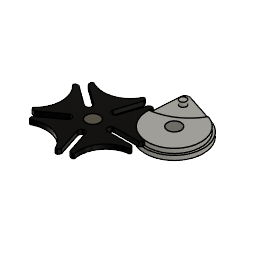
GenevaMechanism (Autodesk Fusion 360 design; units mm, degrees)
part number: 2026-03-22-09-52-00-006
part number: 2026-03-22-09-52-33-959
part number: 2026-03-22-10-12-23-984
part number: 2026-03-22-10-22-25-082
part number: 2026-03-23-03-52-01-189
Autodesk Fusion 360 part; units mm, degrees
sketch "Sketch1" plane through (0, 0, 0) normal (0, 0, 1) x (1, 0, 0) in component "Follower"
  circle A0 centre (0, 0) radius 7.5
  circle A1 centre (0, 0) radius 50
  line L0 (20, -3.75) -> (60, -3.75)
  arc A2 (60, -3.75) -> (60, 3.75) centre (60, 0) ccw
  line L1 (60, 3.75) -> (20, 3.75)
  arc A3 (20, 3.75) -> (20, -3.75) centre (20, 0) ccw
  line L2 (20, 0) -> (60, 0) construction
  line L3 (14.9746, 58.2222) -> (2.6139, 20.1799)
  arc A4 (2.6139, 20.1799) -> (9.7468, 17.8623) centre (6.1803, 19.0211) ccw
  line L4 (9.7468, 17.8623) -> (22.1075, 55.9046)
  arc A5 (22.1075, 55.9046) -> (14.9746, 58.2222) centre (18.541, 57.0634) ccw
  line L5 (-50.7452, 32.2333) -> (-18.3845, 8.7219)
  arc A6 (-18.3845, 8.7219) -> (-13.9761, 14.7895) centre (-16.1803, 11.7557) ccw
  line L6 (-13.9761, 14.7895) -> (-46.3368, 38.3009)
  arc A7 (-46.3368, 38.3009) -> (-50.7452, 32.2333) centre (-48.541, 35.2671) ccw
  line L7 (-46.3368, -38.3009) -> (-13.9761, -14.7895)
  arc A8 (-13.9761, -14.7895) -> (-18.3845, -8.7219) centre (-16.1803, -11.7557) ccw
  line L8 (-18.3845, -8.7219) -> (-50.7452, -32.2333)
  arc A9 (-50.7452, -32.2333) -> (-46.3368, -38.3009) centre (-48.541, -35.2671) ccw
  line L9 (22.1075, -55.9046) -> (9.7468, -17.8623)
  arc A10 (9.7468, -17.8623) -> (2.6139, -20.1799) centre (6.1803, -19.0211) ccw
  line L10 (2.6139, -20.1799) -> (14.9746, -58.2222)
  arc A11 (14.9746, -58.2222) -> (22.1075, -55.9046) centre (18.541, -57.0634) ccw
  circle A12 centre (52.5861, 38.206) radius 30
  line L11 (52.5861, 38.206) -> (20, 0) construction
  line L12 (52.5861, 38.206) -> (6.1803, 19.0211) construction
  circle A13 centre (-20.0861, 61.8187) radius 30
  circle A14 centre (-65, 0) radius 30
  circle A15 centre (-20.0861, -61.8187) radius 30
  circle A16 centre (52.5861, -38.206) radius 30
  dimension "d12" = 15
  dimension "d13" = 100
  dimension "d14" = 7.5
  dimension "d15" = 20
  dimension "d17" = 360
  dimension "d18" = 60
  dimension "d19" = 65
  dimension "d21" = 360
  constraint coincident A0.centre A1.centre
  constraint tangent L0 A2
  constraint tangent A2 L1
  constraint parallel L0 L1
  constraint tangent L1 A3
  constraint tangent L0 A3
  constraint horizontal L2
  constraint horizontal A0.centre A3.centre
  constraint coincident A12.centre L11.start
  constraint coincident A3.centre L2.start
  constraint coincident A4.centre L12.end
  constraint equal L11 L12
  measures "d12" diameter of A0
  measures "d13" diameter of A1
  measures "d14" diameter of A2
  measures "d15" distance of A0.centre A3.centre
  measures "d18" diameter of A12
  measures "d19" distance of A0.centre A12.centre
extrude "Extrude1" add sketch "Sketch1" along normal blind 5 contours A1 L0 L1 A3 L3 A4 L4 L5 A6 L6 L7 A8 L8 L9 A10 L10 A12 A13 A14 A15 A16 makes body 1 in component "Follower"
chamfer "Chamfer1" distance 2.5 angle 45 10 edges at (11.8409, -48.5777, 2.5) (18.9738, -46.2601, 2.5) (-38.1327, -32.3403, 2.5) (-42.5411, -26.2727, 2.5) (-42.5411, 26.2727, 2.5) (-38.1327, 32.3403, 2.5) (11.8409, 48.5777, 2.5) (18.9738, 46.2601, 2.5) (49.8592, -3.75, 2.5) (49.8592, 3.75, 2.5) on bodies 1 in component "Follower"
sketch "Sketch1 (2)" plane through (0, 0, 5) normal (0, 0, 1) x (-1, 0, 0) in component "FollowJoint"
  line L0 (-47.3592, -3.75) -> (-49.6094, -6.2375)
  arc A0 (-49.6094, -6.2375) -> (-49.2915, -8.3875) centre (0, 0) ccw
  arc A1 (-23.2089, -44.2871) -> (-49.2915, -8.3875) centre (-52.5861, -38.206) ccw
  arc A2 (-23.2089, -44.2871) -> (-21.2624, -45.2539) centre (0, 0) ccw
  line L1 (-21.2624, -45.2539) -> (-18.2013, -43.8824)
  line L2 (-18.2013, -43.8824) -> (-9.7468, -17.8623)
  arc A3 (-2.6139, -20.1799) -> (-9.7468, -17.8623) centre (-6.1803, -19.0211) ccw
  line L3 (-2.6139, -20.1799) -> (-11.0683, -46.2001)
  line L4 (-11.0683, -46.2001) -> (-9.3979, -49.1088)
  arc A4 (-9.3979, -49.1088) -> (-7.2549, -49.4709) centre (0, 0) ccw
  arc A5 (34.9476, -35.7584) -> (-7.2549, -49.4709) centre (20.0861, -61.8187) ccw
  arc A6 (34.9476, -35.7584) -> (36.4686, -34.2059) centre (0, 0) ccw
  line L5 (36.4686, -34.2059) -> (36.1102, -30.8708)
  line L6 (36.1102, -30.8708) -> (13.9761, -14.7895)
  arc A7 (18.3845, -8.7219) -> (13.9761, -14.7895) centre (16.1803, -11.7557) ccw
  line L7 (18.3845, -8.7219) -> (40.5186, -24.8032)
  line L8 (40.5186, -24.8032) -> (43.8012, -24.1134)
  arc A8 (43.8012, -24.1134) -> (44.8077, -22.1872) centre (0, 0) ccw
  arc A9 (44.8077, 22.1872) -> (44.8077, -22.1872) centre (65, 0) ccw
  arc A10 (44.8077, 22.1872) -> (43.8012, 24.1134) centre (0, 0) ccw
  line L9 (43.8012, 24.1134) -> (40.5186, 24.8032)
  line L10 (40.5186, 24.8032) -> (18.3845, 8.7219)
  arc A11 (13.9761, 14.7895) -> (18.3845, 8.7219) centre (16.1803, 11.7557) ccw
  line L11 (13.9761, 14.7895) -> (36.1102, 30.8708)
  line L12 (36.1102, 30.8708) -> (36.4686, 34.2059)
  arc A12 (36.4686, 34.2059) -> (34.9476, 35.7584) centre (0, 0) ccw
  arc A13 (-7.2549, 49.4709) -> (34.9476, 35.7584) centre (20.0861, 61.8187) ccw
  arc A14 (-7.2549, 49.4709) -> (-9.3979, 49.1088) centre (0, 0) ccw
  line L13 (-9.3979, 49.1088) -> (-11.0683, 46.2001)
  line L14 (-11.0683, 46.2001) -> (-2.6139, 20.1799)
  arc A15 (-9.7468, 17.8623) -> (-2.6139, 20.1799) centre (-6.1803, 19.0211) ccw
  line L15 (-9.7468, 17.8623) -> (-18.2013, 43.8824)
  line L16 (-18.2013, 43.8824) -> (-21.2624, 45.2539)
  arc A16 (-21.2624, 45.2539) -> (-23.2089, 44.2871) centre (0, 0) ccw
  arc A17 (-49.2915, 8.3875) -> (-23.2089, 44.2871) centre (-52.5861, 38.206) ccw
  arc A18 (-49.2915, 8.3875) -> (-49.6094, 6.2375) centre (0, 0) ccw
  line L17 (-49.6094, 6.2375) -> (-47.3592, 3.75)
  line L18 (-47.3592, 3.75) -> (-20, 3.75)
  arc A19 (-20, -3.75) -> (-20, 3.75) centre (-20, 0) ccw
  line L19 (-20, -3.75) -> (-47.3592, -3.75)
  circle A20 centre (0, 0) radius 7.5
  circle A21 centre (0, 0) radius 7.5
extrude "Extrude1'" add sketch "Sketch1 (2)" against normal blind 10 separate body contours A20 A21 makes body 2 in component "FollowJoint"
sketch "Sketch1 (3)" plane through (0, 0, 0) normal (0, 0, 1) x (1, 0, 0)
sketch "Sketch1 (4)" plane through (0, 0, 0) normal (0, 0, 1) x (1, 0, 0) in component "Cam"
  circle A0 centre (52.5861, 38.206) radius 7.5
  arc A1 (23.2089, 44.2871) -> (49.2915, 8.3875) centre (52.5861, 38.206) ccw
  line L0 (52.5861, 38.206) -> (158.6521, 144.2721) construction
  line L1 (52.5861, 38.206) -> (202.5861, 38.206) construction
  circle A2 centre (79.1026, 64.7225) radius 3.75
  arc A3 (89.365, 69.3879) -> (83.768, 74.985) centre (84.4059, 70.0258) ccw
  line L2 (83.768, 74.985) -> (48.4396, 70.4404)
  line L3 (89.365, 69.3879) -> (84.8205, 34.0595)
  arc A4 (48.6183, 67.9425) -> (82.3226, 34.2382) centre (98.548, 84.168) ccw
  arc A5 (48.6183, 67.9425) -> (82.3226, 34.2382) centre (52.5861, 38.206) ccw
  arc A6 (48.4396, 70.4404) -> (85.0861, 38.206) centre (52.5861, 38.206) ccw
  dimension "d27" = 65
  dimension "d28" = 60
  dimension "d29" = 15
  dimension "d30" = 150
  dimension "d31" = 45
  dimension "d32" = 7.5
  dimension "d33" = 10
  dimension "d34" = 37.5
  dimension "d35" = 45
  dimension "d36" = 105
  dimension "d37" = 65
  constraint concentric A5 A6
  constraint concentric A0 A5
  constraint tangent A1 A5
  constraint horizontal L1
  constraint coincident A0.centre A1.centre
  constraint coincident L0 A2.centre
  constraint coincident L0 A3.centre
  constraint tangent A3 L2
  constraint tangent L2 A6
  constraint tangent A3 L3
  constraint tangent L3 A6
  constraint coincident L3.end A6
  constraint coincident L0 A4.centre
  constraint coincident L1 A6.end
  measures "d27" diameter of A6
  measures "d28" diameter of A5
  measures "d29" diameter of A0
  measures "d30" distance of A0.centre L0.end
  measures "d31" angle of L0 L1
  measures "d32" diameter of A2
  measures "d33" diameter of A3
  measures "d34" distance of A0.centre A2.centre
  measures "d35" distance of A0.centre A3.centre
  measures "d36" diameter of A4
  measures "d37" distance of A0.centre A4.centre
extrude "Extrude1''" add sketch "Sketch1 (4)" along normal blind 5 separate body contours A1 A4 A5 makes body 3 in component "Cam"
extrude "Extrude2" add sketch "Sketch1 (4)" against normal blind 5 contours A3 L2 L3 A6 bodies 3 in component "Cam"
extrude "Extrude3" add sketch "Sketch1 (4)" along normal mid plane 10 contours A2 bodies 3 in component "Cam"
extrude "Extrude1'''" add sketch "Sketch1 (4)" along normal mid plane 10 separate body contours A0 makes body 4 in component "CamJoint"
component "Follower" placed x (1, 0, 0) y (0, 1, 0) z (0, 0, 1) at (0, 0, 0)
component "FollowJoint" placed x (1, 0, 0) y (0, 1, 0) z (0, 0, 1) at (0, 0, 0)
component "Cam" placed x (1, 0, 0) y (0, 1, 0) z (0, 0, 1) at (0, 0, 0)
component "CamJoint" placed x (1, 0, 0) y (0, 1, 0) z (0, 0, 1) at (0, 0, 0)
